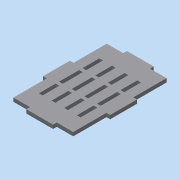
# Autodesk Inventor part: tapadelante
Saved by Autodesk Inventor 2015 (Build 190159000, 159)
## iProperties
Created: 2017-09-28
Part Number: tapadelante
Material: Generic
Document SubType Name: Modeling
Designer: Max
Density: 1 g/cm^3
Appearance: Default
Author: Max
Autodesk Inventor part; units mm, degrees
ref_plane "YZ Plane" through (0, 0, 0) normal (1, 0, 0) x (0, 1, 0)
ref_plane "XZ Plane" through (0, 0, 0) normal (0, 1, 0) x (-1, 0, 0)
ref_plane "XY Plane" through (0, 0, 0) normal (0, 0, 1) x (1, 0, 0)
sketch "Sketch1" plane through (0, 0, 0) normal (0, 0, 1) x (1, 0, 0)
  line L0 (0, 0) -> (89, 0)
  line L1 (89, 0) -> (89, 139)
  line L2 (89, 139) -> (0, 139)
  line L3 (0, 139) -> (0, 0)
  line L4 (24.5, 0) -> (64.5, 0)
  line L5 (64.5, 0) -> (64.5, -5.5)
  line L6 (64.5, -5.5) -> (24.5, -5.5)
  line L7 (24.5, -5.5) -> (24.5, 0)
  line L8 (24.5, 139) -> (64.5, 139)
  line L9 (64.5, 139) -> (64.5, 144.5)
  line L10 (64.5, 144.5) -> (24.5, 144.5)
  line L11 (24.5, 144.5) -> (24.5, 139)
  line L12 (0, 49.5) -> (-5.5, 49.5)
  line L13 (-5.5, 49.5) -> (-5.5, 89.5)
  line L14 (-5.5, 89.5) -> (0, 89.5)
  line L15 (0, 89.5) -> (0, 49.5)
  line L16 (89, 49.5) -> (94.5, 49.5)
  line L17 (94.5, 49.5) -> (94.5, 89.5)
  line L18 (94.5, 89.5) -> (89, 89.5)
  line L19 (89, 89.5) -> (89, 49.5)
  dimension "d5" = 89
  dimension "d6" = 139
  dimension "d7" = 40
  dimension "d8" = 5.5
  dimension "d9" = 40
  dimension "d10" = 5.5
  dimension "d11" = 5.5
  dimension "d12" = 40
  dimension "d13" = 5.5
  dimension "d14" = 40
  constraints: 40 end point, 10 parallel, 5 horizontal, 5 perpendicular, 4 point on line
  measures "d5" distance of L2.end L1.end
  measures "d6" distance of L1.end L0.end
  measures "d7" distance of L5.end L6.end
  measures "d8" distance of L4.end L5.end
  measures "d9" distance of L10.end L9.end
  measures "d10" distance of L9.end L8.end
  measures "d11" distance of L13.end L14.end
  measures "d12" distance of L12.end L13.end
  measures "d13" distance of L18.end L17.end
  measures "d14" distance of L17.end L16.end
extrude "Extrusion1" add sketch "Sketch1" along normal blind 5.5
sketch "Sketch2" plane through (0, 0, 5.5) normal (0, 0, 1) x (1, 0, 0)
  line L0 (64.5, 144.5) -> (24.5, 144.5) projected
  line L1 (13.48, 54.5) -> (18.88, 54.5)
  line L2 (18.88, 54.5) -> (18.88, 84.5)
  line L3 (18.88, 84.5) -> (13.48, 84.5)
  line L4 (13.48, 84.5) -> (13.48, 54.5)
  line L5 (32.36, 84.5) -> (37.76, 84.5)
  line L6 (37.76, 84.5) -> (37.76, 54.5)
  line L7 (37.76, 54.5) -> (32.36, 54.5)
  line L8 (32.36, 54.5) -> (32.36, 84.5)
  line L9 (51.24, 84.5) -> (56.64, 84.5)
  line L10 (56.64, 84.5) -> (56.64, 54.5)
  line L11 (56.64, 54.5) -> (51.24, 54.5)
  line L12 (51.24, 54.5) -> (51.24, 84.5)
  line L13 (70.12, 84.5) -> (75.52, 84.5)
  line L14 (75.52, 84.5) -> (75.52, 54.5)
  line L15 (75.52, 54.5) -> (70.12, 54.5)
  line L16 (70.12, 54.5) -> (70.12, 84.5)
  line L17 (13.48, 89.5) -> (18.88, 89.5)
  line L18 (18.88, 89.5) -> (18.88, 114.5)
  line L19 (18.88, 114.5) -> (13.48, 114.5)
  line L20 (13.48, 114.5) -> (13.48, 89.5)
  line L21 (37.76, 114.5) -> (32.36, 114.5)
  line L22 (32.36, 114.5) -> (32.36, 89.5)
  line L23 (32.36, 89.5) -> (37.76, 89.5)
  line L24 (37.76, 89.5) -> (37.76, 114.5)
  line L25 (51.24, 114.5) -> (56.64, 114.5)
  line L26 (56.64, 114.5) -> (56.64, 89.5)
  line L27 (56.64, 89.5) -> (51.24, 89.5)
  line L28 (51.24, 89.5) -> (51.24, 114.5)
  line L29 (70.12, 89.5) -> (75.52, 89.5)
  line L30 (75.52, 89.5) -> (75.52, 114.5)
  line L31 (75.52, 114.5) -> (70.12, 114.5)
  line L32 (70.12, 114.5) -> (70.12, 89.5)
  line L33 (-5.5, 89.5) -> (-5.5, 49.5) projected
  line L34 (94.5, 49.5) -> (94.5, 89.5) projected
  line L35 (13.48, 49.5) -> (18.88, 49.5)
  line L36 (18.88, 49.5) -> (18.88, 24.5)
  line L37 (18.88, 24.5) -> (13.48, 24.5)
  line L38 (13.48, 24.5) -> (13.48, 49.5)
  line L39 (37.76, 24.5) -> (32.36, 24.5)
  line L40 (32.36, 24.5) -> (32.36, 49.5)
  line L41 (32.36, 49.5) -> (37.76, 49.5)
  line L42 (37.76, 49.5) -> (37.76, 24.5)
  line L43 (51.24, 24.5) -> (56.64, 24.5)
  line L44 (56.64, 24.5) -> (56.64, 49.5)
  line L45 (56.64, 49.5) -> (51.24, 49.5)
  line L46 (51.24, 49.5) -> (51.24, 24.5)
  line L47 (70.12, 49.5) -> (75.52, 49.5)
  line L48 (75.52, 49.5) -> (75.52, 24.5)
  line L49 (75.52, 24.5) -> (70.12, 24.5)
  line L50 (70.12, 24.5) -> (70.12, 49.5)
  point P0 (0, 0)
  dimension "d24" = 30
  dimension "d25" = 25
  constraints: 96 end point, 16 parallel, 14 point on line, 8 horizontal, 8 perpendicular
  measures "d24" distance of L2.end L1.end
  measures "d25" distance of L18.end L17.end
extrude "Extrusion2" cut sketch "Sketch2" against normal blind 10
body "Solid1"
